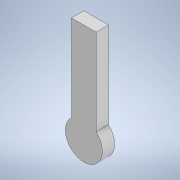
# Autodesk Inventor part: Throttle Arm
Saved by Autodesk Inventor 2020.4 (Build 244396000, 396)
## iProperties
Created: 2022-04-15
Part Number: Throttle Arm
Material: Generic
Document SubType Name: Modeling
Designer: Gurkin
Density: 1 g/cm^3
Appearance: Default
Author: Gurkin
Autodesk Inventor part; units mm, degrees
ref_plane "YZ Plane" through (0, 0, 0) normal (1, 0, 0) x (0, 1, 0)
ref_plane "XZ Plane" through (0, 0, 0) normal (0, 1, 0) x (-1, 0, 0)
ref_plane "XY Plane" through (0, 0, 0) normal (0, 0, 1) x (1, 0, 0)
sketch "Sketch1" plane through (0, 0, 0) normal (0, 0, 1) x (1, 0, 0)
  line L0 (-20, 162.3607) -> (20, 162.3607)
  line L1 (-20, 22.3607) -> (-20, 162.3607)
  line L2 (20, 162.3607) -> (20, 22.3607)
  arc A0 (-20, 22.3607) -> (20, 22.3607) centre (0, 0) ccw
  dimension "d16" = 40
  dimension "d19" = 140
  dimension "d53" = 30
  constraints: 6 end point, 2 parallel, 2 point on circle, 1 centre point, 1 coincident, 1 horizontal, 1 perpendicular
  measures "d16" distance between parallel lines of L2 L1
  measures "d19" distance of L1.start L0.start
  measures "d53" radius of A0
extrude "Extrusion1" add sketch "Sketch1" along normal blind 20
sketch "Sketch10" plane through (0, 0, 0) normal (0, 0, -1) x (-1, 0, 0)
  circle A0 centre (0, 0) radius 8
  dimension "d54" = 16
  constraints: 1 centre point, 1 coincident
  measures "d54" diameter of A0
extrude "Extrusion7" cut sketch "Sketch10" against normal blind 10
body "Solid1"
